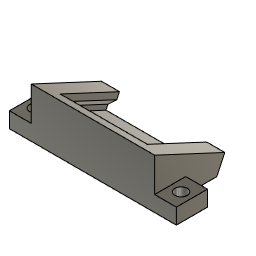
Fysetc_5i_LCD (Autodesk Fusion 360 archive; units mm, degrees)
design "Fysetc_5i_LCD_Mount"
Autodesk Fusion 360 part; units mm, degrees
sketch "Sketch1" plane through (0, 0, 0) normal (0, 1, 0) x (1, 0, 0)
  line L0 (0, 0) -> (40, 0)
  line L1 (40, 0) -> (40, -5)
  line L2 (40, -5) -> (0, -5)
  line L3 (0, -5) -> (0, 0)
  line L4 (40, 0) -> (52, 0)
  line L5 (52, 0) -> (52, -16.5)
  line L6 (52, -16.5) -> (40, -16.5)
  line L7 (40, -16.5) -> (40, 0)
  line L8 (0, 0) -> (-12, 0)
  line L9 (-12, 0) -> (-12, -16.5)
  line L10 (-12, -16.5) -> (0, -16.5)
  line L11 (0, -16.5) -> (0, 0)
  dimension "d1" = 40
  dimension "d2" = 5
  dimension "d3" = 12
  dimension "d4" = 12
  dimension "d5" = 16.5
  constraint horizontal L0
  constraint vertical L1
  constraint horizontal L2
  constraint vertical L3
  constraint coincident L0.start L3.end
  constraint horizontal L4
  constraint vertical L5
  constraint horizontal L6
  constraint vertical L7
  constraint horizontal L8
  constraint vertical L9
  constraint horizontal L10
  constraint vertical L11
  constraint coincident L6.end L10
  measures "d1" distance of L0.start L0.end
  measures "d2" distance of L0.end L1.end
  measures "d3" distance of L0.end L4.end
  measures "d4" distance of L0.start L8.end
  measures "d5" distance of L4.end L5.end
  measures "d10" distance of L0.start
extrude "Extrude1" add sketch "Sketch1" along normal blind 10
sketch "Sketch2" plane through (0, 0, 0) normal (0, 0, -1) x (1, 0, 0)
  line L0 (52, 0) -> (-12, 0)
  line L1 (-12, 0) -> (-12, -10)
  line L2 (-12, -10) -> (52, -10)
  line L3 (52, -10) -> (52, 0)
  line L4 (-12, -5) -> (52, -5) construction
  circle A0 centre (44.75, -5) radius 2
  circle A1 centre (-4.75, -5) radius 2
  dimension "d8" = 4
  dimension "d9" = 4
  dimension "d10" = 49.5
  dimension "d11" = 69
  dimension "d12" = 7.25
  constraint midpoint L1 L4.start
  constraint midpoint L3 L4.end
  constraint coincident L4 A0.centre
  constraint coincident L4 A1.centre
  measures "d8" diameter of A0
  measures "d9" diameter of A1
  measures "d10" distance of A0.centre A1.centre
  measures "d12" distance of L4.start A1.centre
extrude "Extrude2" cut sketch "Sketch2" against normal blind 6 contours A0 | A1
fillet "Fillet1" radius 5 4 edges at (46, 10, 16.5) (46, 0, 16.5) (-6, 0, 16.5) (-6, 10, 16.5)
sketch "Sketch3" plane through (-12, 0, 0) normal (-1, 0, 0) x (0, -1, 0)
  arc A0 (0, 11.5) -> (-10, 11.5) centre (-5, 11.5) ccw
  line L0 (-10, 11.5) -> (-10, 0)
  line L1 (-10, 0) -> (0, 0)
  line L2 (0, 0) -> (0, 11.5)
  circle A1 centre (-5, 11.5) radius 2
  dimension "d16" = 4
  constraint concentric A0 A1
  measures "d16" diameter of A1
extrude "Extrude3" cut sketch "Sketch3" against normal blind 66 contours A1
sketch "Sketch4" plane through (-12, 0, 0) normal (-1, 0, 0) x (0, -1, 0)
  circle A0 centre (-5, 11.5) radius 2
  arc A1 (0, 11.5) -> (-10, 11.5) centre (-5, 11.5) ccw
  line L0 (-10, 11.5) -> (-10, 0)
  line L1 (-10, 0) -> (0, 0)
  line L2 (0, 0) -> (0, 11.5)
  circle A2 centre (-5, 11.5) radius 3.25
  dimension "d19" = 6.5
  constraint concentric A0 A2
  measures "d19" diameter of A2
extrude "Extrude4" cut sketch "Sketch4" against normal blind 6 contours A2
sketch "Sketch5" plane through (52, 0, 0) normal (1, 0, 0) x (0, 1, 0)
  circle A0 centre (5, 11.5) radius 2
  arc A1 (10, 11.5) -> (0, 11.5) centre (5, 11.5) ccw
  line L0 (0, 11.5) -> (0, 0)
  line L1 (0, 0) -> (10, 0)
  line L2 (10, 0) -> (10, 11.5)
  line L3 (7.9, 13.1743) -> (5, 14.8486)
  line L4 (5, 14.8486) -> (2.1, 13.1743)
  line L5 (2.1, 13.1743) -> (2.1, 9.8257)
  line L6 (2.1, 9.8257) -> (5, 8.1514)
  line L7 (5, 8.1514) -> (7.9, 9.8257)
  line L8 (7.9, 9.8257) -> (7.9, 13.1743)
  point P0 (5, 11.5)
  dimension "d22" = 5.8
  constraint coincident P0 A0.centre
  measures "d22" distance of L5 L8
extrude "Extrude5" cut sketch "Sketch5" against normal blind 3.5 contours L3 L4 L5 L6 L7 L8
sketch "Sketch6" plane through (0, 0, 0) normal (1, 0, 0) x (0, 1, 0)
  circle A0 centre (5, 11.5) radius 2
  arc A1 (10, 11.5) -> (0, 11.5) centre (5, 11.5) ccw
  line L0 (0, 11.5) -> (0, 5)
  line L1 (0, 5) -> (10, 5)
  line L2 (10, 5) -> (10, 11.5)
extrude "Extrude6" cut sketch "Sketch6" along normal through all and the other way through all contours A0 | A1 L0 L1 L2
extrude "Extrude7" add sketch "Sketch6" along normal blind 40
sketch "Sketch7" plane through (0, 0, 5) normal (0, 0, 1) x (-1, 0, 0)
  circle A0 centre (4.75, -5) radius 2
  line L0 (0, 0) -> (0, -10)
  line L1 (0, -10) -> (12, -10)
  line L2 (12, -10) -> (12, 0)
  line L3 (12, 0) -> (0, 0)
  line L4 (-40, -10) -> (-40, 0)
  line L5 (-40, 0) -> (-52, 0)
  line L6 (-52, 0) -> (-52, -10)
  line L7 (-52, -10) -> (-40, -10)
  circle A1 centre (-44.75, -5) radius 2
  circle A2 centre (4.75, -5) radius 3
  circle A3 centre (-44.75, -5) radius 3
  line L8 (-52, -10) -> (-49.5, -10)
  line L9 (-49.5, -10) -> (-49.5, 0)
  line L10 (-49.5, 0) -> (-52, 0)
  line L11 (-52, 0) -> (-52, -10)
  line L12 (12, -10) -> (9.5, -10)
  line L13 (9.5, -10) -> (9.5, 0)
  line L14 (9.5, 0) -> (12, 0)
  line L15 (12, 0) -> (12, -10)
  dimension "d28" = 6
  dimension "d29" = 6
  dimension "d30" = 4.75
  dimension "d31" = 4.75
  constraint concentric A0 A2
  constraint concentric A1 A3
  constraint horizontal L8
  constraint vertical L9
  constraint horizontal L10
  constraint vertical L11
  constraint coincident L6.end L7.start
  constraint horizontal L12
  constraint vertical L13
  constraint horizontal L14
  constraint vertical L15
  constraint coincident L3 L13.end
  constraint coincident L1.end L2.start
  measures "d28" diameter of A2
  measures "d29" diameter of A3
  measures "d30" distance of A0.centre L13
  measures "d31" distance of A1.centre L9
extrude "Extrude8" cut sketch "Sketch7" against normal blind 6 contours L1 L2 L3 L12 L13 L14 L15 | L5 L6 L7 L8 L9 L10 L11
sketch "Sketch8" plane through (0, 0, 0) normal (0, 0, -1) x (1, 0, 0)
  line L0 (49.5, -10) -> (49.5, 0)
  line L1 (49.5, 0) -> (-9.5, 0)
  line L2 (-9.5, 0) -> (-9.5, -10)
  line L3 (-9.5, -10) -> (49.5, -10)
  circle A0 centre (-4.75, -5) radius 2
  circle A1 centre (44.75, -5) radius 2
  circle A2 centre (44.75, -5) radius 1.65
  circle A3 centre (-4.75, -5) radius 1.65
  dimension "d36" = 3.3
  dimension "d37" = 3.3
  constraint concentric A1 A2
  constraint concentric A0 A3
  measures "d36" diameter of A2
  measures "d37" diameter of A3
extrude "Extrude10" add sketch "Sketch8" against normal up to surface (5 mm away) contours A0 | A1
sketch "Sketch9" plane through (0, 0, 0) normal (0, 0, -1) x (1, 0, 0)
  circle A0 centre (44.75, -5) radius 1.65
  circle A1 centre (-4.75, -5) radius 1.65
  line L0 (49.5, -10) -> (49.5, 0)
  line L1 (49.5, 0) -> (-9.5, 0)
  line L2 (-9.5, 0) -> (-9.5, -10)
  line L3 (-9.5, -10) -> (49.5, -10)
  circle A2 centre (44.75, -5) radius 1.8
  circle A3 centre (-4.75, -5) radius 1.8
  dimension "d41" = 3.6
  dimension "d42" = 3.6
  constraint concentric A0 A2
  constraint concentric A1 A3
  measures "d41" diameter of A2
  measures "d42" diameter of A3
extrude "Extrude11" cut sketch "Sketch9" against normal blind 6 contours A2 | A3
extrude "Extrude12" cut 1 faces at (40, 5.0498, 6.5019) along direction (-1, 0, 0) blind 0.2
extrude "Extrude13" cut 1 faces at (0, 5.0498, 6.5019) along direction (1, 0, 0) blind 0.2
sketch "Sketch10" plane through (0.2, 0, 0) normal (-1, 0, 0) x (0, -1, 0)
  circle A0 centre (-5, 11.5) radius 2
  line L0 (-10, 11.5) -> (-10, 5)
  line L1 (-10, 5) -> (0, 5)
  line L2 (0, 5) -> (0, 11.5)
  arc A1 (0, 11.5) -> (-10, 11.5) centre (-5, 11.5) ccw
  line L3 (-10, 0) -> (0, 0)
  line L4 (0, 0) -> (0, 5)
  line L5 (0, 5) -> (-10, 5)
  line L6 (-10, 5) -> (-10, 0)
  line L7 (-10, 0) -> (-20, 0)
  line L8 (-22.5357, 5.4378) -> (0, 15.9464)
  line L9 (-22.5357, 5.4378) -> (-20, 0)
  line L10 (0, 11.5) -> (0, 15.9464)
  dimension "d50" = 6
  dimension "d51" = 10
  dimension "d56" = 25
  constraint coincident L3.start L6.end
  constraint perpendicular L6 L7
  constraint coincident L2 L8.end
  constraint coincident L7 L9.end
  constraint perpendicular L8 L9
  constraint coincident L7.end L9.end
  constraint coincident L2.end A1.start
  measures "d50" distance of L7.end L8.start
  measures "d51" distance of L3.start L7.end
  measures "d56" angle of L7 L8
extrude "Extrude14" add sketch "Sketch10" against normal up to surface (39.6 mm away) contours A0 L8 | A1 L8 L10 | L0 L6 L7 L8 L9 picked at (-5.9137, 12.0616)
extrude "Extrude15" cut sketch "Sketch10" against normal blind 71 contours A0 L0 A1 L8
sketch "Sketch11" plane through (0, 16.4279, -7.6604) normal (0, 0.906308, -0.422618) x (-1, 0, 0)
  line L0 (-39.8, 14.4524) -> (-39.8, 8.4524)
  line L1 (-39.8, 8.4524) -> (-0.2, 8.4524)
  line L2 (-0.2, 8.4524) -> (-0.2, 14.4524)
  line L3 (-0.2, 14.4524) -> (-39.8, 14.4524)
  line L4 (-4, 14.4524) -> (-36, 14.4524)
  line L5 (-36, 14.4524) -> (-36, 8.9524)
  line L6 (-36, 8.9524) -> (-4, 8.9524)
  line L7 (-4, 8.9524) -> (-4, 14.4524)
  line L8 (-6, 14.4524) -> (-34, 14.4524)
  line L9 (-34, 14.4524) -> (-34, 10.4524)
  line L10 (-34, 10.4524) -> (-6, 10.4524)
  line L11 (-6, 10.4524) -> (-6, 14.4524)
  line L12 (-6, 10.4524) -> (-4, 10.4524)
  line L13 (-4, 10.4524) -> (-4, 8.9524)
  line L14 (-4, 8.9524) -> (-6, 8.9524)
  line L15 (-6, 8.9524) -> (-6, 10.4524)
  line L16 (-34, 10.4524) -> (-36, 10.4524)
  line L17 (-36, 10.4524) -> (-36, 8.9524)
  line L18 (-36, 8.9524) -> (-34, 8.9524)
  line L19 (-34, 8.9524) -> (-34, 10.4524)
  dimension "d57" = 5.5
  dimension "d58" = 32
  dimension "d59" = 39.6
  dimension "d60" = 3.8
  dimension "d61" = 28
  dimension "d62" = 4
  dimension "d63" = 2
  constraint horizontal L4
  constraint vertical L5
  constraint horizontal L6
  constraint vertical L7
  constraint coincident L3 L4.start
  constraint horizontal L8
  constraint vertical L9
  constraint horizontal L10
  constraint vertical L11
  constraint coincident L4 L8.start
  constraint horizontal L12
  constraint vertical L13
  constraint horizontal L14
  constraint vertical L15
  constraint horizontal L16
  constraint vertical L17
  constraint horizontal L18
  constraint vertical L19
  measures "d57" distance of L4.end L5.end
  measures "d58" distance of L5.end L6.end
  measures "d59" distance of L0.end L1.end
  measures "d60" distance of L0 L5
  measures "d61" distance of L8.start L8.end
  measures "d62" distance of L8.start L10.end
  measures "d63" distance of L7 L11
extrude "Extrude16" cut sketch "Sketch11" against normal blind 21 contours L3 L4 L8 L9 L10 L11 | L5 L6 L16 L17 L18 L19 | L6 L10 L15 L19 | L6 L7 L12 L13 L14 L15
chamfer "Chamfer2" distance 2 angle 45 2 edges at (6, 11.329, 6.2501) (34, 11.329, 6.2501)
sketch "Sketch12" plane through (0, 0, 5) normal (0, 0, 1) x (-1, 0, 0)
  circle A0 centre (4.75, -5) radius 1.8
  line L0 (9.5, -10) -> (9.5, 0)
  line L1 (9.5, 0) -> (-0.2, 0)
  line L2 (-0.2, 0) -> (-0.2, -10)
  line L3 (-0.2, -10) -> (9.5, -10)
  line L4 (-49.5, 0) -> (-39.8, 0)
  circle A1 centre (-44.75, -5) radius 1.8
  line L5 (-49.5, 0) -> (-49.5, -10)
  line L6 (-49.5, -10) -> (-39.8, -10)
  line L7 (-39.8, -10) -> (-39.8, 0)
  line L8 (-39.8, 0) -> (-49.5, 0)
  line L9 (9.5, -10) -> (9.5, 0)
extrude "Extrude17" add sketch "Sketch12" against normal up to surface (5 mm away) contours A0 | A1
sketch "Sketch13" plane through (0, 0, 5) normal (0, 0, 1) x (-1, 0, 0)
  line L0 (9.5, -10) -> (9.5, 0)
  line L1 (9.5, 0) -> (-0.2, 0)
  line L2 (-0.2, 0) -> (-0.2, -10)
  line L3 (-0.2, -10) -> (9.5, -10)
  line L4 (-49.5, 0) -> (-49.5, -10)
  line L5 (-49.5, -10) -> (-39.8, -10)
  line L6 (-39.8, -10) -> (-39.8, 0)
  line L7 (-39.8, 0) -> (-49.5, 0)
  line L8 (-39.8, -5) -> (-43.3, -5) construction
  line L9 (-0.2, -5) -> (3.3, -5) construction
  circle A0 centre (-43.3, -5) radius 2
  circle A1 centre (3.3, -5) radius 2
  line L10 (9.5, -10) -> (6.8, -10)
  line L11 (6.8, -10) -> (6.8, 0)
  line L12 (6.8, 0) -> (9.5, 0)
  line L13 (9.5, 0) -> (9.5, -10)
  line L14 (-49.5, -10) -> (-46.8, -10)
  line L15 (-46.8, -10) -> (-46.8, 0)
  line L16 (-46.8, 0) -> (-49.5, 0)
  line L17 (-49.5, 0) -> (-49.5, -10)
  dimension "d70" = 3.5
  dimension "d71" = 3.5
  dimension "d72" = 4
  dimension "d73" = 4
  dimension "d74" = 3.5
  dimension "d75" = 3.5
  constraint midpoint L6 L8.start
  constraint perpendicular L4 L8
  constraint midpoint L2 L9.start
  constraint perpendicular L2 L9
  constraint coincident L8.end A0.centre
  constraint coincident L9.end A1.centre
  constraint horizontal L10
  constraint vertical L11
  constraint horizontal L12
  constraint vertical L13
  constraint coincident L1 L11.end
  constraint coincident L0.start L3.end
  constraint horizontal L14
  constraint vertical L15
  constraint horizontal L16
  constraint vertical L17
  constraint coincident L7 L15.end
  constraint coincident L4.end L5.start
  measures "d70" distance of L8.start L8.end
  measures "d71" distance of L9.start L9.end
  measures "d72" diameter of A0
  measures "d73" diameter of A1
  measures "d74" distance of L8.end L15
  measures "d75" distance of L9.end L11
extrude "Extrude18" cut sketch "Sketch13" against normal blind 6 contours L0 L1 L3 L10 L11 L12 L13 | L4 L5 L7 L14 L15 L16 L17 | A0 | A1
equation "d4 = d3"
equation "d9 = d8"
equation "d12 = ( 64.00 mm - d10 ) / 2"
equation "d31 = d30"
equation "d60 = ( 39.60 mm - d58 ) / 2"
equation "d63 = ( d58 - d61 ) / 2"
equation "d70 = d71"
equation "d74 = d70"
equation "d75 = d71"

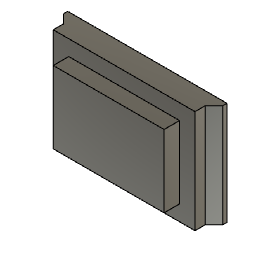
design "Fysetc_5i_LCD_Mount_Back"
Autodesk Fusion 360 part; units mm, degrees
sketch "Sketch1" plane through (0, 0, 0) normal (0, 1, 0) x (1, 0, 0)
  line L0 (0, 0) -> (127.4, 0) construction
  line L1 (127.4, 0) -> (127.4, -76.2) construction
  line L2 (127.4, -76.2) -> (0, -76.2) construction
  line L3 (0, -76.2) -> (0, 0) construction
  circle A0 centre (0, -76.2) radius 2
  circle A1 centre (127.4, -76.2) radius 2
  circle A2 centre (127.4, 0) radius 2
  circle A3 centre (0, 0) radius 2
  line L4 (2.2, -76.7) -> (125.2, -76.7)
  line L5 (125.2, -76.7) -> (125.2, 3)
  line L6 (125.2, 3) -> (2.2, 3)
  line L7 (2.2, 3) -> (2.2, -76.7)
  line L8 (-11.8, -80.45) -> (135.2, -80.45)
  line L9 (135.2, -80.45) -> (135.2, 4)
  line L10 (135.2, 4) -> (-11.8, 4)
  line L11 (-11.8, 4) -> (-11.8, -80.45)
  line L12 (137.2, 6) -> (-13.8, 6)
  line L13 (-13.8, 6) -> (-13.8, -82.45)
  line L14 (-13.8, -82.45) -> (137.2, -82.45)
  line L15 (137.2, -82.45) -> (137.2, 6)
  line L16 (8.4, -74.8) -> (120, -74.8)
  line L17 (120, -74.8) -> (120, -5.9)
  line L18 (120, -5.9) -> (8.4, -5.9)
  line L19 (8.4, -5.9) -> (8.4, -74.8)
  dimension "d1" = 76.2
  dimension "d2" = 127.4
  dimension "d3" = 4
  dimension "d4" = 4
  dimension "d5" = 4
  dimension "d6" = 4
  dimension "d8" = 123
  dimension "d9" = 0.5
  dimension "d10" = 3
  dimension "d11" = 2.2
  dimension "d12" = 3.75
  dimension "d13" = 1
  dimension "d14" = 14
  dimension "d15" = 10
  dimension "d16" = 2
  dimension "d22" = 1.9
  dimension "d23" = 8.9
  dimension "d24" = 6.2
  dimension "d25" = 5.2
  constraint horizontal L0
  constraint vertical L1
  constraint horizontal L2
  constraint vertical L3
  constraint coincident L0.start L3.end
  constraint coincident L2.end L3.start
  constraint coincident L1.end L2.start
  constraint coincident L0.end L1.start
  constraint horizontal L4
  constraint vertical L5
  constraint horizontal L6
  constraint vertical L7
  constraint horizontal L8
  constraint vertical L9
  constraint horizontal L10
  constraint vertical L11
  constraint horizontal L16
  constraint vertical L17
  constraint horizontal L18
  constraint vertical L19
  measures "d1" distance of L0.start L2.end
  measures "d2" distance of L0.start L0.end
  measures "d3" diameter of A0
  measures "d4" diameter of A1
  measures "d5" diameter of A2
  measures "d6" diameter of A3
  measures "d8" distance of L4.start L4.end
  measures "d9" distance of L2.end L4
  measures "d10" distance of L0.start L6
  measures "d11" distance of L0.start L7
  measures "d12" distance of L4 L8
  measures "d13" distance of L6 L10
  measures "d14" distance of L7 L11
  measures "d15" distance of L5 L9
  measures "d22" distance of L4 L16
  measures "d23" distance of L6 L18
  measures "d24" distance of L7 L19
  measures "d25" distance of L5 L17
extrude "Extrude1" add sketch "Sketch1" along normal blind 3 contours L4 L5 L6 L7 | L8 L9 L10 L11 | L16 L17 L18 L19
sketch "Sketch2" plane through (0, 0, 0) normal (0, -1, 0) x (1, 0, 0)
  circle A0 centre (0, 0) radius 2
  circle A1 centre (127.4, 76.2) radius 2
  circle A2 centre (127.4, 0) radius 2
  circle A3 centre (0, 76.2) radius 2
  line L0 (-11.8, 80.45) -> (-11.8, -4)
  line L1 (-11.8, -4) -> (135.2, -4)
  line L2 (135.2, -4) -> (135.2, 80.45)
  line L3 (135.2, 80.45) -> (-11.8, 80.45)
  line L4 (-11.3, -3.5) -> (134.7, -3.5)
  line L5 (134.7, -3.5) -> (134.7, 79.95)
  line L6 (134.7, 79.95) -> (-11.3, 79.95)
  line L7 (-11.3, 79.95) -> (-11.3, -3.5)
  circle A4 centre (0, 76.2) radius 3.75
  circle A5 centre (0, 0) radius 3.5
  circle A6 centre (127.4, 0) radius 3.5
  circle A7 centre (127.4, 76.2) radius 3.75
  dimension "d29" = -0.5
  constraint concentric A3 A4
  constraint concentric A0 A5
  constraint concentric A2 A6
  constraint concentric A1 A7
  constraint tangent L6 A4
  constraint tangent L6 A7
  constraint tangent L4 A6
  constraint tangent L4 A5
extrude "Extrude4" add sketch "Sketch2" along normal blind 6 contours A5 | A6 | A7 | A4
fillet "Fillet2" radius 3 4 edges at (-11.8, 1.5, -4) (-11.8, 1.5, 80.45) (135.2, 1.5, -4) (135.2, 1.5, 80.45)
sketch "Sketch3" plane through (0, 0, 0) normal (0, -1, 0) x (1, 0, 0)
  arc A0 (135.2, 77.45) -> (132.2, 80.45) centre (132.2, 77.45) ccw
  line L0 (132.2, 80.45) -> (-8.8, 80.45)
  arc A1 (-8.8, 80.45) -> (-11.8, 77.45) centre (-8.8, 77.45) ccw
  line L1 (-11.8, 77.45) -> (-11.8, -1)
  arc A2 (-11.8, -1) -> (-8.8, -4) centre (-8.8, -1) ccw
  line L2 (-8.8, -4) -> (132.2, -4)
  arc A3 (132.2, -4) -> (135.2, -1) centre (132.2, -1) ccw
  line L3 (135.2, -1) -> (135.2, 77.45)
  circle A4 centre (0, 0) radius 3.5
  circle A5 centre (0, 76.2) radius 3.75
  circle A6 centre (127.4, 0) radius 3.5
  circle A7 centre (127.4, 76.2) radius 3.75
  line L4 (30.2, -0.6) -> (4.2, -0.6)
  line L5 (4.2, -0.6) -> (4.2, 15.4)
  line L6 (4.2, 15.4) -> (30.2, 15.4)
  line L7 (30.2, 15.4) -> (30.2, -0.6)
  line L8 (-11.8, 19) -> (-2.8, 19)
  line L9 (-2.8, 19) -> (-2.8, 35)
  line L10 (-2.8, 35) -> (-11.8, 35)
  line L11 (-11.8, 35) -> (-11.8, 19)
  line L12 (23.4, 32.5) -> (2.4, 32.5)
  line L13 (2.4, 32.5) -> (2.4, 41.5)
  line L14 (2.4, 41.5) -> (23.4, 41.5)
  line L15 (23.4, 41.5) -> (23.4, 32.5)
  line L16 (86.45, 38.225) -> (36.95, 38.225) construction
  circle A8 centre (36.95, 38.225) radius 1.5
  circle A9 centre (86.45, 38.225) radius 1.5
  dimension "d33" = 26
  dimension "d34" = 16
  dimension "d35" = 3.4
  dimension "d36" = 4.2
  dimension "d37" = 23
  dimension "d38" = 16
  dimension "d39" = 9
  dimension "d40" = 36.5
  dimension "d41" = 14.2
  dimension "d42" = 21
  dimension "d43" = 9
  dimension "d44" = 49.5
  dimension "d45" = 3
  dimension "d46" = 3
  dimension "d47" = 84.45
  dimension "d48" = 42.225
  dimension "d49" = 147
  dimension "d50" = 48.75
  constraint horizontal L4
  constraint vertical L5
  constraint horizontal L6
  constraint vertical L7
  constraint horizontal L8
  constraint vertical L9
  constraint horizontal L10
  constraint vertical L11
  constraint coincident L1 L8.start
  constraint horizontal L12
  constraint vertical L13
  constraint horizontal L14
  constraint vertical L15
  constraint horizontal L16
  constraint coincident L16.end A8.centre
  constraint coincident L16.start A9.centre
  measures "d33" distance of L4.start L4.end
  measures "d34" distance of L4.start L6.end
  measures "d35" distance of L2 L4
  measures "d36" distance of A4.centre L5
  measures "d37" distance of L2 L8
  measures "d38" distance of L8.end L9.end
  measures "d39" distance of L8.start L8.end
  measures "d40" distance of L2 L12
  measures "d41" distance of L1 L13
  measures "d42" distance of L12.start L12.end
  measures "d43" distance of L12.start L14.end
  measures "d44" distance of L16.start L16.end
  measures "d45" diameter of A8
  measures "d46" diameter of A9
  measures "d47" distance of L0 L2
  measures "d48" distance of L0 L16
  measures "d49" distance of L1 L3
  measures "d50" distance of L3 L16.start
extrude "Extrude5" cut sketch "Sketch3" against normal through all contours L1 L8 L9 L10 L11 | L4 L5 L6 L7 | L12 L13 L14 L15
sketch "Sketch4" plane through (0, 3, 0) normal (0, 1, 0) x (-1, 0, 0)
  line L0 (2.8, 35) -> (11.8, 35)
  line L1 (11.8, 35) -> (11.8, 77.45)
  arc A0 (11.8, 77.45) -> (8.8, 80.45) centre (8.8, 77.45) ccw
  line L2 (8.8, 80.45) -> (-132.2, 80.45)
  arc A1 (-132.2, 80.45) -> (-135.2, 77.45) centre (-132.2, 77.45) ccw
  line L3 (-135.2, 77.45) -> (-135.2, -1)
  arc A2 (-135.2, -1) -> (-132.2, -4) centre (-132.2, -1) ccw
  line L4 (-132.2, -4) -> (8.8, -4)
  arc A3 (8.8, -4) -> (11.8, -1) centre (8.8, -1) ccw
  line L5 (11.8, -1) -> (11.8, 19)
  line L6 (11.8, 19) -> (2.8, 19)
  line L7 (2.8, 19) -> (2.8, 35)
  line L8 (-4.2, 15.4) -> (-4.2, -0.6)
  line L9 (-4.2, -0.6) -> (-30.2, -0.6)
  line L10 (-30.2, -0.6) -> (-30.2, 15.4)
  line L11 (-30.2, 15.4) -> (-4.2, 15.4)
  line L12 (-2.4, 41.5) -> (-2.4, 32.5)
  line L13 (-2.4, 32.5) -> (-23.4, 32.5)
  line L14 (-23.4, 32.5) -> (-23.4, 41.5)
  line L15 (-23.4, 41.5) -> (-2.4, 41.5)
  circle A4 centre (0, 0) radius 2
  circle A5 centre (-127.4, 76.2) radius 2
  circle A6 centre (-127.4, 0) radius 2
  circle A7 centre (0, 76.2) radius 2
  line L16 (-75.45, 48.225) -> (-47.95, 48.225)
  line L17 (-47.95, 48.225) -> (-47.95, 28.225)
  line L18 (-47.95, 28.225) -> (-75.45, 28.225)
  line L19 (-75.45, 28.225) -> (-75.45, 48.225)
  constraint horizontal L16
  constraint vertical L17
  constraint horizontal L18
  constraint vertical L19
extrude "Extrude6" add sketch "Sketch4" along normal blind 2 contours L16 L17 L18 L19
sketch "Sketch5" plane through (0, 5, 0) normal (0, 1, 0) x (-1, 0, 0)
  line L0 (-75.45, 28.225) -> (-47.95, 28.225)
  line L1 (-47.95, 28.225) -> (-47.95, 48.225)
  line L2 (-47.95, 48.225) -> (-75.45, 48.225)
  line L3 (-75.45, 48.225) -> (-75.45, 28.225)
  line L4 (-47.95, 48.225) -> (-46.25, 48.225)
  line L5 (-46.25, 48.225) -> (-46.25, 28.225)
  line L6 (-46.25, 28.225) -> (-47.95, 28.225)
  line L7 (-47.95, 28.225) -> (-47.95, 48.225)
  line L8 (-75.45, 48.225) -> (-77.15, 48.225)
  line L9 (-77.15, 48.225) -> (-77.15, 28.225)
  line L10 (-77.15, 28.225) -> (-75.45, 28.225)
  line L11 (-75.45, 28.225) -> (-75.45, 48.225)
  dimension "d59" = 1.7
  dimension "d60" = 1.7
  constraint horizontal L4
  constraint vertical L5
  constraint horizontal L6
  constraint vertical L7
  constraint coincident L1.end L2.start
  constraint coincident L0.end L6
  constraint horizontal L8
  constraint vertical L9
  constraint horizontal L10
  constraint vertical L11
  constraint coincident L2.end L3.start
  constraint coincident L0.start L10
  measures "d59" distance of L2.end L8.end
  measures "d60" distance of L1.end L4.end
extrude "Extrude7" add sketch "Sketch5" along normal blind 2.5
chamfer "Chamfer2" distance 1.7 angle 45 2 edges at (46.25, 5, 38.225) (77.15, 5, 38.225)
sketch "Sketch6" plane through (0, 3, 0) normal (0, 1, 0) x (-1, 0, 0)
  line L0 (-75.45, 28.225) -> (-75.45, 48.225)
  line L1 (-75.45, 48.225) -> (-47.95, 48.225)
  line L2 (-47.95, 48.225) -> (-47.95, 28.225)
  line L3 (-47.95, 28.225) -> (-75.45, 28.225)
  line L4 (2.8, 35) -> (11.8, 35)
  line L5 (11.8, 35) -> (11.8, 77.45)
  arc A0 (11.8, 77.45) -> (8.8, 80.45) centre (8.8, 77.45) ccw
  line L6 (8.8, 80.45) -> (-132.2, 80.45)
  arc A1 (-132.2, 80.45) -> (-135.2, 77.45) centre (-132.2, 77.45) ccw
  line L7 (-135.2, 77.45) -> (-135.2, -1)
  arc A2 (-135.2, -1) -> (-132.2, -4) centre (-132.2, -1) ccw
  line L8 (-132.2, -4) -> (8.8, -4)
  arc A3 (8.8, -4) -> (11.8, -1) centre (8.8, -1) ccw
  line L9 (11.8, -1) -> (11.8, 19)
  line L10 (11.8, 19) -> (2.8, 19)
  line L11 (2.8, 19) -> (2.8, 35)
  line L12 (-23.4, 32.5) -> (-23.4, 41.5)
  line L13 (-23.4, 41.5) -> (-2.4, 41.5)
  line L14 (-2.4, 41.5) -> (-2.4, 32.5)
  line L15 (-2.4, 32.5) -> (-23.4, 32.5)
  line L16 (-30.2, -0.6) -> (-30.2, 15.4)
  line L17 (-30.2, 15.4) -> (-4.2, 15.4)
  line L18 (-4.2, 15.4) -> (-4.2, -0.6)
  line L19 (-4.2, -0.6) -> (-30.2, -0.6)
  circle A4 centre (0, 0) radius 2
  circle A5 centre (-127.4, 76.2) radius 2
  circle A6 centre (-127.4, 0) radius 2
  circle A7 centre (0, 76.2) radius 2
extrude "Extrude8" cut sketch "Sketch6" against normal blind 55
sketch "Sketch7" plane through (0, 0, 0) normal (0, -1, 0) x (1, 0, 0)
  line L0 (47.95, 28.225) -> (75.45, 28.225)
  line L1 (75.45, 28.225) -> (75.45, 48.225)
  line L2 (75.45, 48.225) -> (47.95, 48.225)
  line L3 (47.95, 48.225) -> (47.95, 28.225)
  line L4 (50.95, 31.225) -> (72.45, 31.225)
  line L5 (72.45, 31.225) -> (72.45, 45.225)
  line L6 (72.45, 45.225) -> (50.95, 45.225)
  line L7 (50.95, 45.225) -> (50.95, 31.225)
  dimension "d66" = -3
extrude "Extrude9" cut sketch "Sketch7" against normal blind 3
equation "d48 = 84.45 mm / 2"
equation "d50 = ( 147.00 mm - d44 ) / 2"
equation "d60 = d59"

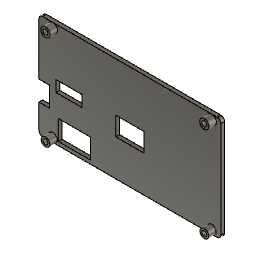
design "Fysetc_5i_LCD_Back"
Autodesk Fusion 360 part; units mm, degrees
sketch "Sketch1" plane through (0, 0, 0) normal (0, 1, 0) x (1, 0, 0)
  line L0 (0, 0) -> (127.4, 0) construction
  line L1 (127.4, 0) -> (127.4, -76.2) construction
  line L2 (127.4, -76.2) -> (0, -76.2) construction
  line L3 (0, -76.2) -> (0, 0) construction
  circle A0 centre (0, -76.2) radius 2
  circle A1 centre (127.4, -76.2) radius 2
  circle A2 centre (127.4, 0) radius 2
  circle A3 centre (0, 0) radius 2
  line L4 (2.2, -76.7) -> (125.2, -76.7)
  line L5 (125.2, -76.7) -> (125.2, 3)
  line L6 (125.2, 3) -> (2.2, 3)
  line L7 (2.2, 3) -> (2.2, -76.7)
  line L8 (-11.8, -80.45) -> (135.2, -80.45)
  line L9 (135.2, -80.45) -> (135.2, 4)
  line L10 (135.2, 4) -> (-11.8, 4)
  line L11 (-11.8, 4) -> (-11.8, -80.45)
  line L12 (137.2, 6) -> (-13.8, 6)
  line L13 (-13.8, 6) -> (-13.8, -82.45)
  line L14 (-13.8, -82.45) -> (137.2, -82.45)
  line L15 (137.2, -82.45) -> (137.2, 6)
  line L16 (8.4, -74.8) -> (120, -74.8)
  line L17 (120, -74.8) -> (120, -5.9)
  line L18 (120, -5.9) -> (8.4, -5.9)
  line L19 (8.4, -5.9) -> (8.4, -74.8)
  dimension "d1" = 76.2
  dimension "d2" = 127.4
  dimension "d3" = 4
  dimension "d4" = 4
  dimension "d5" = 4
  dimension "d6" = 4
  dimension "d8" = 123
  dimension "d9" = 0.5
  dimension "d10" = 3
  dimension "d11" = 2.2
  dimension "d12" = 3.75
  dimension "d13" = 1
  dimension "d14" = 14
  dimension "d15" = 10
  dimension "d16" = 2
  dimension "d22" = 1.9
  dimension "d23" = 8.9
  dimension "d24" = 6.2
  dimension "d25" = 5.2
  constraint horizontal L0
  constraint vertical L1
  constraint horizontal L2
  constraint vertical L3
  constraint coincident L0.start L3.end
  constraint coincident L2.end L3.start
  constraint coincident L1.end L2.start
  constraint coincident L0.end L1.start
  constraint horizontal L4
  constraint vertical L5
  constraint horizontal L6
  constraint vertical L7
  constraint horizontal L8
  constraint vertical L9
  constraint horizontal L10
  constraint vertical L11
  constraint horizontal L16
  constraint vertical L17
  constraint horizontal L18
  constraint vertical L19
  measures "d1" distance of L0.start L2.end
  measures "d2" distance of L0.start L0.end
  measures "d3" diameter of A0
  measures "d4" diameter of A1
  measures "d5" diameter of A2
  measures "d6" diameter of A3
  measures "d8" distance of L4.start L4.end
  measures "d9" distance of L2.end L4
  measures "d10" distance of L0.start L6
  measures "d11" distance of L0.start L7
  measures "d12" distance of L4 L8
  measures "d13" distance of L6 L10
  measures "d14" distance of L7 L11
  measures "d15" distance of L5 L9
  measures "d22" distance of L4 L16
  measures "d23" distance of L6 L18
  measures "d24" distance of L7 L19
  measures "d25" distance of L5 L17
extrude "Extrude1" add sketch "Sketch1" along normal blind 3 contours L4 L5 L6 L7 | L8 L9 L10 L11 | L16 L17 L18 L19
sketch "Sketch2" plane through (0, 0, 0) normal (0, -1, 0) x (1, 0, 0)
  circle A0 centre (0, 0) radius 2
  circle A1 centre (127.4, 76.2) radius 2
  circle A2 centre (127.4, 0) radius 2
  circle A3 centre (0, 76.2) radius 2
  line L0 (-11.8, 80.45) -> (-11.8, -4)
  line L1 (-11.8, -4) -> (135.2, -4)
  line L2 (135.2, -4) -> (135.2, 80.45)
  line L3 (135.2, 80.45) -> (-11.8, 80.45)
  line L4 (-11.3, -3.5) -> (134.7, -3.5)
  line L5 (134.7, -3.5) -> (134.7, 79.95)
  line L6 (134.7, 79.95) -> (-11.3, 79.95)
  line L7 (-11.3, 79.95) -> (-11.3, -3.5)
  circle A4 centre (0, 76.2) radius 3.75
  circle A5 centre (0, 0) radius 3.5
  circle A6 centre (127.4, 0) radius 3.5
  circle A7 centre (127.4, 76.2) radius 3.75
  dimension "d29" = -0.5
  constraint concentric A3 A4
  constraint concentric A0 A5
  constraint concentric A2 A6
  constraint concentric A1 A7
  constraint tangent L6 A4
  constraint tangent L6 A7
  constraint tangent L4 A6
  constraint tangent L4 A5
extrude "Extrude4" add sketch "Sketch2" along normal blind 6 contours A5 | A6 | A7 | A4
extrude "Extrude12" cut sketch "Sketch2" against normal blind 6 contours L0 L1 L2 L3
fillet "Fillet2" radius 3 4 edges at (-11.3, 1.5, -3.5) (134.7, 1.5, -3.5) (134.7, 1.5, 79.95) (-11.3, 1.5, 79.95)
sketch "Sketch3" plane through (0, 0, 0) normal (0, -1, 0) x (1, 0, 0)
  circle A0 centre (0, 0) radius 3.5
  circle A1 centre (0, 76.2) radius 3.75
  circle A2 centre (127.4, 0) radius 3.5
  circle A3 centre (127.4, 76.2) radius 3.75
  line L0 (30.2, -0.6) -> (4.2, -0.6)
  line L1 (4.2, -0.6) -> (4.2, 15.4)
  line L2 (4.2, 15.4) -> (30.2, 15.4)
  line L3 (30.2, 15.4) -> (30.2, -0.6)
  line L4 (-11.8, 19) -> (-2.8, 19)
  line L5 (-2.8, 19) -> (-2.8, 35)
  line L6 (-2.8, 35) -> (-11.8, 35)
  line L7 (-11.8, 35) -> (-11.8, 19)
  line L8 (23.4, 32.5) -> (2.4, 32.5)
  line L9 (2.4, 32.5) -> (2.4, 41.5)
  line L10 (2.4, 41.5) -> (23.4, 41.5)
  line L11 (23.4, 41.5) -> (23.4, 32.5)
  line L12 (86.45, 38.225) -> (36.95, 38.225) construction
  circle A4 centre (36.95, 38.225) radius 1.5
  circle A5 centre (86.45, 38.225) radius 1.5
  line L13 (-8.3, -3.5) -> (0, -3.5)
  line L14 (134.7, -0.5) -> (134.7, 76.95)
  line L15 (131.7, 79.95) -> (127.4, 79.95)
  line L16 (127.4, 79.95) -> (0, 79.95)
  line L17 (-11.3, 76.95) -> (-11.3, -0.5)
  arc A6 (-8.3, 79.95) -> (-11.3, 76.95) centre (-8.3, 76.95) ccw
  arc A7 (-11.3, -0.5) -> (-8.3, -3.5) centre (-8.3, -0.5) ccw
  line L18 (0, -3.5) -> (127.4, -3.5)
  line L19 (127.4, -3.5) -> (131.7, -3.5)
  arc A8 (131.7, -3.5) -> (134.7, -0.5) centre (131.7, -0.5) ccw
  arc A9 (134.7, 76.95) -> (131.7, 79.95) centre (131.7, 76.95) ccw
  line L20 (0, 79.95) -> (-8.3, 79.95)
  dimension "d33" = 26
  dimension "d34" = 16
  dimension "d36" = 4.2
  dimension "d38" = 16
  dimension "d39" = 9
  dimension "d42" = 21
  dimension "d43" = 9
  dimension "d44" = 49.5
  dimension "d45" = 3
  dimension "d46" = 3
  constraint horizontal L0
  constraint vertical L1
  constraint horizontal L2
  constraint vertical L3
  constraint horizontal L4
  constraint vertical L5
  constraint horizontal L6
  constraint vertical L7
  constraint horizontal L8
  constraint vertical L9
  constraint horizontal L10
  constraint vertical L11
  constraint horizontal L12
  constraint coincident L12.end A4.centre
  constraint coincident L12.start A5.centre
  measures "d33" distance of L0.start L0.end
  measures "d34" distance of L0.start L2.end
  measures "d36" distance of A0.centre L1
  measures "d38" distance of L4.end L5.end
  measures "d39" distance of L4.start L4.end
  measures "d42" distance of L8.start L8.end
  measures "d43" distance of L8.start L10.end
  measures "d44" distance of L12.start L12.end
  measures "d45" diameter of A4
  measures "d46" diameter of A5
extrude "Extrude5" cut sketch "Sketch3" against normal through all contours L4 L5 L6 L17 | L4 L6 L7 L17 | L0 L1 L2 L3 | L8 L9 L10 L11
sketch "Sketch4" plane through (0, 3, 0) normal (0, 1, 0) x (-1, 0, 0)
  line L0 (2.8, 35) -> (11.3, 35)
  line L1 (11.3, 19) -> (2.8, 19)
  line L2 (2.8, 19) -> (2.8, 35)
  line L3 (-4.2, 15.4) -> (-4.2, -0.6)
  line L4 (-4.2, -0.6) -> (-30.2, -0.6)
  line L5 (-30.2, -0.6) -> (-30.2, 15.4)
  line L6 (-30.2, 15.4) -> (-4.2, 15.4)
  line L7 (-2.4, 41.5) -> (-2.4, 32.5)
  line L8 (-2.4, 32.5) -> (-23.4, 32.5)
  line L9 (-23.4, 32.5) -> (-23.4, 41.5)
  line L10 (-23.4, 41.5) -> (-2.4, 41.5)
  circle A0 centre (0, 0) radius 2
  circle A1 centre (-127.4, 76.2) radius 2
  circle A2 centre (-127.4, 0) radius 2
  circle A3 centre (0, 76.2) radius 2
  line L11 (-75.45, 48.225) -> (-47.95, 48.225)
  line L12 (-47.95, 48.225) -> (-47.95, 28.225)
  line L13 (-47.95, 28.225) -> (-75.45, 28.225)
  line L14 (-75.45, 28.225) -> (-75.45, 48.225)
  line L15 (11.3, 35) -> (11.3, 76.95)
  line L16 (8.3, 79.95) -> (-131.7, 79.95)
  line L17 (-134.7, 76.95) -> (-134.7, -0.5)
  line L18 (-131.7, -3.5) -> (8.3, -3.5)
  arc A4 (11.3, 76.95) -> (8.3, 79.95) centre (8.3, 76.95) ccw
  arc A5 (-131.7, 79.95) -> (-134.7, 76.95) centre (-131.7, 76.95) ccw
  arc A6 (-134.7, -0.5) -> (-131.7, -3.5) centre (-131.7, -0.5) ccw
  arc A7 (8.3, -3.5) -> (11.3, -0.5) centre (8.3, -0.5) ccw
  line L19 (11.3, -0.5) -> (11.3, 19)
  constraint horizontal L11
  constraint vertical L12
  constraint horizontal L13
  constraint vertical L14
extrude "Extrude6" add sketch "Sketch4" along normal blind 2 contours L11 L12 L13 L14
sketch "Sketch5" plane through (0, 5, 0) normal (0, 1, 0) x (-1, 0, 0)
  line L0 (-75.45, 28.225) -> (-47.95, 28.225)
  line L1 (-47.95, 28.225) -> (-47.95, 48.225)
  line L2 (-47.95, 48.225) -> (-75.45, 48.225)
  line L3 (-75.45, 48.225) -> (-75.45, 28.225)
  line L4 (-47.95, 48.225) -> (-45.95, 48.225)
  line L5 (-45.95, 48.225) -> (-45.95, 28.225)
  line L6 (-45.95, 28.225) -> (-47.95, 28.225)
  line L7 (-47.95, 28.225) -> (-47.95, 48.225)
  line L8 (-75.45, 48.225) -> (-77.45, 48.225)
  line L9 (-77.45, 48.225) -> (-77.45, 28.225)
  line L10 (-77.45, 28.225) -> (-75.45, 28.225)
  line L11 (-75.45, 28.225) -> (-75.45, 48.225)
  dimension "d59" = 2
  dimension "d60" = 2
  constraint horizontal L4
  constraint vertical L5
  constraint horizontal L6
  constraint vertical L7
  constraint coincident L1.end L2.start
  constraint coincident L0.end L6
  constraint horizontal L8
  constraint vertical L9
  constraint horizontal L10
  constraint vertical L11
  constraint coincident L2.end L3.start
  constraint coincident L0.start L10
  measures "d59" distance of L2.end L8.end
  measures "d60" distance of L1.end L4.end
extrude "Extrude7" add sketch "Sketch5" along normal blind 3
chamfer "Chamfer2" distance 2 angle 45 2 edges at (45.95, 5, 38.225) (77.45, 5, 38.225)
sketch "Sketch8" plane through (0, 3, 0) normal (0, 1, 0) x (-1, 0, 0)
  line L0 (-75.45, 28.225) -> (-75.45, 48.225)
  line L1 (-75.45, 48.225) -> (-47.95, 48.225)
  line L2 (-47.95, 48.225) -> (-47.95, 28.225)
  line L3 (-47.95, 28.225) -> (-75.45, 28.225)
  line L4 (2.8, 35) -> (11.3, 35)
  line L5 (11.3, 19) -> (2.8, 19)
  line L6 (2.8, 19) -> (2.8, 35)
  line L7 (-23.4, 32.5) -> (-23.4, 41.5)
  line L8 (-23.4, 41.5) -> (-2.4, 41.5)
  line L9 (-2.4, 41.5) -> (-2.4, 32.5)
  line L10 (-2.4, 32.5) -> (-23.4, 32.5)
  line L11 (-30.2, -0.6) -> (-30.2, 15.4)
  line L12 (-30.2, 15.4) -> (-4.2, 15.4)
  line L13 (-4.2, 15.4) -> (-4.2, -0.6)
  line L14 (-4.2, -0.6) -> (-30.2, -0.6)
  circle A0 centre (0, 0) radius 2
  circle A1 centre (-127.4, 76.2) radius 2
  circle A2 centre (-127.4, 0) radius 2
  circle A3 centre (0, 76.2) radius 2
  line L15 (-50.45, 30.725) -> (-72.95, 30.725)
  line L16 (-72.95, 30.725) -> (-72.95, 45.725)
  line L17 (-72.95, 45.725) -> (-50.45, 45.725)
  line L18 (-50.45, 45.725) -> (-50.45, 30.725)
  line L19 (11.3, 35) -> (11.3, 76.95)
  line L20 (8.3, 79.95) -> (-131.7, 79.95)
  line L21 (-134.7, 76.95) -> (-134.7, -0.5)
  line L22 (-131.7, -3.5) -> (8.3, -3.5)
  arc A4 (11.3, 76.95) -> (8.3, 79.95) centre (8.3, 76.95) ccw
  arc A5 (-131.7, 79.95) -> (-134.7, 76.95) centre (-131.7, 76.95) ccw
  arc A6 (-134.7, -0.5) -> (-131.7, -3.5) centre (-131.7, -0.5) ccw
  arc A7 (8.3, -3.5) -> (11.3, -0.5) centre (8.3, -0.5) ccw
  line L23 (11.3, -0.5) -> (11.3, 19)
  dimension "d69" = 2.5
extrude "Extrude10" cut sketch "Sketch8" along normal blind 5 contours L0 L1 L2 L3 | L4 L5 L6 L19 L20 L21 L22 A4 A5 A6 A7 L23 | L15 L16 L17 L18
extrude "Extrude11" cut sketch "Sketch8" against normal blind 6 contours L15 L16 L17 L18
sketch "Sketch9" plane through (0, 0, 0) normal (0, -1, 0) x (1, 0, 0)
  line L0 (72.95, 45.725) -> (72.95, 30.725)
  line L1 (72.95, 30.725) -> (50.45, 30.725)
  line L2 (50.45, 30.725) -> (50.45, 45.725)
  line L3 (50.45, 45.725) -> (72.95, 45.725)
  line L4 (-11.3, 35) -> (-2.8, 35)
  line L5 (-2.8, 35) -> (-2.8, 19)
  line L6 (-2.8, 19) -> (-11.3, 19)
  line L7 (-11.3, 19) -> (-11.3, -0.5)
  arc A0 (-11.3, -0.5) -> (-8.3, -3.5) centre (-8.3, -0.5) ccw
  line L8 (-8.3, -3.5) -> (0, -3.5)
  circle A1 centre (0, 0) radius 3.5
  line L9 (0, -3.5) -> (127.4, -3.5)
  circle A2 centre (127.4, 0) radius 3.5
  line L10 (127.4, -3.5) -> (131.7, -3.5)
  arc A3 (131.7, -3.5) -> (134.7, -0.5) centre (131.7, -0.5) ccw
  line L11 (134.7, -0.5) -> (134.7, 76.95)
  arc A4 (134.7, 76.95) -> (131.7, 79.95) centre (131.7, 76.95) ccw
  line L12 (131.7, 79.95) -> (127.4, 79.95)
  circle A5 centre (127.4, 76.2) radius 3.75
  line L13 (127.4, 79.95) -> (0, 79.95)
  circle A6 centre (0, 76.2) radius 3.75
  line L14 (0, 79.95) -> (-8.3, 79.95)
  arc A7 (-8.3, 79.95) -> (-11.3, 76.95) centre (-8.3, 76.95) ccw
  line L15 (-11.3, 76.95) -> (-11.3, 35)
  line L16 (30.2, 15.4) -> (30.2, -0.6)
  line L17 (30.2, -0.6) -> (4.2, -0.6)
  line L18 (4.2, -0.6) -> (4.2, 15.4)
  line L19 (4.2, 15.4) -> (30.2, 15.4)
  line L20 (23.4, 41.5) -> (23.4, 32.5)
  line L21 (23.4, 32.5) -> (2.4, 32.5)
  line L22 (2.4, 32.5) -> (2.4, 41.5)
  line L23 (2.4, 41.5) -> (23.4, 41.5)
  line L24 (50.45, 30.725) -> (72.95, 30.725)
  line L25 (72.95, 30.725) -> (72.95, 25.725)
  line L26 (72.95, 25.725) -> (50.45, 25.725)
  line L27 (50.45, 25.725) -> (50.45, 30.725)
  line L28 (50.45, 45.725) -> (72.95, 45.725)
  line L29 (72.95, 45.725) -> (72.95, 40.725)
  line L30 (72.95, 40.725) -> (50.45, 40.725)
  line L31 (50.45, 40.725) -> (50.45, 45.725)
  dimension "d77" = 5
  dimension "d78" = 5
  constraint horizontal L24
  constraint vertical L25
  constraint horizontal L26
  constraint vertical L27
  constraint coincident L1.end L2.start
  constraint horizontal L28
  constraint vertical L29
  constraint horizontal L30
  constraint vertical L31
  constraint coincident L2.end L3.start
  constraint coincident L0.start L29
  constraint coincident L0.end L25
  measures "d77" distance of L0.start L29.end
  measures "d78" distance of L1.end L26.end
extrude "Extrude13" cut sketch "Sketch9" against normal blind 6 contours L1 L24 L25 L26 L27
extrude "Extrude14" add sketch "Sketch9" against normal up to surface (3 mm away) contours L0 L2 L3 L28 L29 L30 L31
equation "d60 = d59"
equation "d78 = d77"
